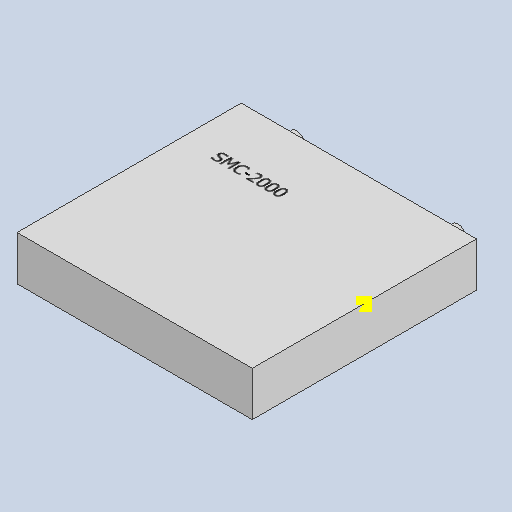
# Autodesk Inventor part: SMC-2000(GPS_BOARD)
Saved by Autodesk Inventor 2025.2 (Build 292293000, 293)
## iProperties
Created: 2025-07-30
Part Number: SMC-2000(GPS_BOARD)
Material: 일반
Document SubType Name: Modeling
Designer: jbhma
Density: 1 g/cm^3
Appearance: 기본값
Author: jbhma
Autodesk Inventor part; units mm, degrees
ref_plane "YZ Plane" through (0, 0, 0) normal (1, 0, 0) x (0, 1, 0)
ref_plane "XZ Plane" through (0, 0, 0) normal (0, 1, 0) x (-1, 0, 0)
ref_plane "XY Plane" through (0, 0, 0) normal (0, 0, 1) x (1, 0, 0)
sketch "스케치1" plane through (0, 0, 0) normal (0, 1, 0) x (-1, 0, 0)
  line L0 (63.5, 30.25) -> (0, 30.25)
  line L1 (0, 30.25) -> (0, -30.25)
  line L2 (0, -30.25) -> (63.5, -30.25)
  line L3 (63.5, -30.25) -> (63.5, 30.25)
  point P0 (0, 0)
  point P1 (0, 0)
  dimension "d0" = 63.5
  dimension "d1" = 60.5
  constraints: 8 end point, 2 parallel, 1 coincident, 1 horizontal, 1 midpoint, 1 perpendicular
  measures "d0" distance of L2.end L1.end
  measures "d1" distance of L1.end L0.end
extrude "돌출1" add sketch "스케치1" along normal blind 12
sketch "스케치3" plane through (0, 0, -30.25) normal (0, 0, -1) x (-1, 0, 0)
  line L0 (0, 0) -> (63.5, 0) projected
  line L1 (63.5, 0) -> (63.5, 12) projected
  line L2 (0, 12) -> (63.5, 12) projected
  line L3 (0, 0) -> (0, 12) projected
  circle A0 centre (10, 6) radius 2
  circle A1 centre (53.5, 6) radius 2
  point P0 (0, 0)
  dimension "d4" = 4
  dimension "d5" = 10
  dimension "d6" = 10
  constraints: 2 centre point
  measures "d4" diameter of A0
  measures "d5" distance from line of L3 A0.centre
  measures "d6" distance from line of L1 A1.centre
extrude "돌출2" add sketch "스케치3" along normal blind 5 contours A0 | A1
sketch "스케치4" plane through (0, 12, 0) normal (0, 1, 0) x (1, 0, 0)
  line L0 (-54.9197, 16.2745) -> (-7.8987, 16.2745) construction
  line L1 (-7.8987, 16.2745) -> (-7.8987, 0.7952) construction
  line L2 (-7.8987, 0.7952) -> (-54.9197, 0.7952) construction
  line L3 (-54.9197, 0.7952) -> (-54.9197, 16.2745) construction
  point P0 (0, 0)
  constraints: 2 other
